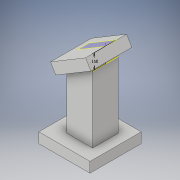
# Autodesk Inventor part: Plaque
Saved by Autodesk Inventor 2018 (Build 220112000, 112)
## iProperties
Created: 2019-03-11
Part Number: Plaque
Material: Generic
Document SubType Name: Modeling
Designer: 871357
Density: 1 g/cm^3
Appearance: Default
Author: 871357
Autodesk Inventor part; units mm, degrees
ref_plane "YZ Plane" through (0, 0, 0) normal (1, 0, 0) x (0, 1, 0)
ref_plane "XZ Plane" through (0, 0, 0) normal (0, 1, 0) x (-1, 0, 0)
ref_plane "XY Plane" through (0, 0, 0) normal (0, 0, 1) x (1, 0, 0)
sketch "Sketch1" plane through (0, 0, 0) normal (0, 1, 0) x (-1, 0, 0)
  line L0 (-1.4187, 3.9318) -> (11.2813, 3.9318)
  line L1 (11.2813, 3.9318) -> (11.2813, -8.7682)
  line L2 (11.2813, -8.7682) -> (-1.4187, -8.7682)
  line L3 (-1.4187, -8.7682) -> (-1.4187, 3.9318)
  point P0 (0, 0)
  dimension "d0" = 12.7
  dimension "d1" = 12.7
  constraints: 8 end point, 2 parallel, 1 horizontal, 1 perpendicular
  measures "d0" distance of L1.end L2.end
  measures "d1" distance of L0.end L1.end
extrude "Extrusion1" add sketch "Sketch1" along normal blind 2.54
sketch "Sketch2" plane through (0, 2.54, 0) normal (0, 1, 0) x (1, 0, 0)
  line L0 (-1.1213, -0.7568) -> (-7.4713, -0.7568)
  line L1 (-7.4713, -0.7568) -> (-7.4713, 5.5932)
  line L2 (-7.4713, 5.5932) -> (-1.1213, 5.5932)
  line L3 (-1.1213, 5.5932) -> (-1.1213, -0.7568)
  line L4 (1.4187, 8.7682) -> (-11.2813, 8.7682) projected
  line L5 (1.4187, -3.9318) -> (1.4187, 8.7682) projected
  point P0 (0, 0)
  dimension "d4" = 6.35
  dimension "d5" = 6.35
  dimension "d6" = 3.175
  dimension "d7" = 2.54
  constraints: 8 end point, 2 parallel, 1 horizontal, 1 perpendicular
  measures "d4" distance of L1.end L2.end
  measures "d5" distance of L0.end L1.end
  measures "d6" distance between parallel lines of L4 L2
  measures "d7" distance between parallel lines of L5 L3
extrude "Extrusion2" add sketch "Sketch2" along normal blind 16.51
sketch "Sketch3" plane through (-1.1213, 2.54, 0.7568) normal (1, 0, 0) x (0, 0, -1)
  line L0 (0, 16.51) -> (6.35, 16.51) projected
  line L1 (3.175, 16.51) -> (3.175, 20.32)
  line L2 (3.175, 20.32) -> (5.6637, 20.32)
  point P0 (0.7568, -2.54)
  dimension "d10" = 3.81
  constraints: 4 end point, 2 coincident, 1 midpoint, 1 perpendicular, 1 vertical
  measures "d10" distance of L1.start L1.end
ref_plane "Work Plane1" through (-1.1213, 22.86, -4.9069) normal (0.5144958, -0.8574929, 0) x (0, 0, 1)
sketch "Sketch4" plane through (-1.1213, 22.86, -4.9069) normal (0.5144958, -0.8574929, 0) x (0, 0, 1)
  line L0 (-2.5913, 9.9453) -> (7.5687, 9.9453)
  line L1 (7.5687, 9.9453) -> (7.5687, -0.2147)
  line L2 (7.5687, -0.2147) -> (-2.5913, -0.2147)
  line L3 (-2.5913, -0.2147) -> (-2.5913, 9.9453)
  line L4 (5.6637, 7.4053) -> (5.6637, 1.9602) projected
  line L5 (-0.6863, 7.4053) -> (5.6637, 7.4053) projected
  point P0 (4.9069, 10.7999)
  dimension "d11" = 10.16
  dimension "d12" = 10.16
  dimension "d13" = 1.905
  dimension "d14" = 2.54
  constraints: 8 end point, 2 parallel, 1 horizontal, 1 perpendicular
  measures "d11" distance of L1.end L2.end
  measures "d12" distance of L0.end L1.end
  measures "d13" distance between parallel lines of L4 L1
  measures "d14" distance between parallel lines of L5 L0
extrude "Extrusion3" add sketch "Sketch4" along normal blind 2.54
sketch "Sketch5" plane through (0, 19.05, 0) normal (0, 1, 0) x (1, 0, 0)
  line L0 (-8.3425, -2.6618) -> (-8.3425, 7.4982) projected
  line L1 (-8.3425, 7.4982) -> (0.3696, 7.4982) projected
  line L2 (0.3696, 7.4982) -> (0.3696, -2.6618) projected
  line L3 (0.3696, -2.6618) -> (-8.3425, -2.6618) projected
  line L4 (-7.4713, -0.7568) -> (-7.4713, 5.5932) projected
  line L5 (-2.5344, -0.7568) -> (-7.4713, -0.7568) projected
  line L6 (-2.5344, 5.5932) -> (-2.5344, -0.7568) projected
  line L7 (-7.4713, 5.5932) -> (-2.5344, 5.5932) projected
  line L8 (-1.1213, -0.7568) -> (-2.5344, -0.7568)
  line L9 (-2.5344, -0.7568) -> (-2.5344, 5.5932)
  line L10 (-2.5344, 5.5932) -> (-1.1213, 5.5932)
  line L11 (-1.1213, 5.5932) -> (-1.1213, -0.7568)
  point P0 (0, 0)
  constraints: 8 end point, 2 parallel, 1 horizontal, 1 perpendicular
extrude "Extrusion4" add sketch "Sketch5" along normal up to next contours L6 L10 L11 L8
body "Solid1"
